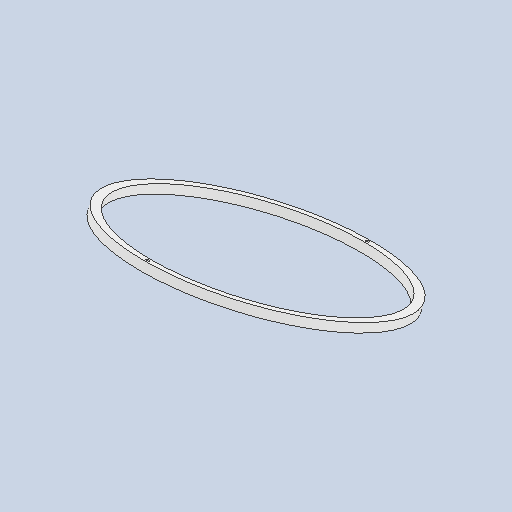
# Autodesk Inventor part: belt_liner_v2_Pom_r
Saved by Autodesk Inventor 2025.2 (Build 292293000, 293)
## iProperties
Created: 2025-01-06
Part Number: belt_liner_v2_Pom_r
Material: ABS プラスチック
Document SubType Name: Modeling
Designer: haruy
Density: 1.06 g/cm^3
Appearance: 白
Author: haruy
Autodesk Inventor part; units mm, degrees
ref_plane "YZ Plane" through (0, 0, 0) normal (1, 0, 0) x (0, 1, 0)
ref_plane "XZ Plane" through (0, 0, 0) normal (0, 1, 0) x (-1, 0, 0)
ref_plane "XY Plane" through (0, 0, 0) normal (0, 0, 1) x (1, 0, 0)
derived "belt_liner_v2_Sketch_Base.ipt"
sketch "スケッチ1" plane through (300, 0, 0) normal (1, 0, 0) x (0, 1, 0)
  circle A0 centre (0, 0) radius 23.875
  circle A1 centre (981.994578, -416.831968) radius 23.875 construction
  line L0 (0, 0) -> (0, -985.832038)
  line L1 (0.888552, 67.547515) -> (6.749519, 81.355087)
  line L2 (6.749519, 81.355087) -> (503.82214, -129.639722)
  line L3 (503.82214, -129.639722) -> (497.961173, -143.447295)
  line L4 (497.961173, -143.447295) -> (0.888552, 67.547515)
  line L5 (0, 0) -> (981.994578, -416.831968)
  line L6 (-41.329946, -31.913035) -> (-47.190913, -45.720608)
  line L7 (-47.190913, -45.720608) -> (953.397863, -470.445344)
  line L8 (953.397863, -470.445344) -> (959.258829, -456.637772)
  line L9 (959.258829, -456.637772) -> (-41.329946, -31.913035)
  line L10 (11.023029, 79.54109) -> (11.023029, 79.54109)
  line L11 (0.888552, 67.547515) -> (82.443045, 32.929686)
  line L12 (82.443045, 32.929686) -> (80.489389, 28.327162)
  line L13 (80.489389, 28.327162) -> (-1.065103, 62.94499)
  line L14 (-1.065103, 62.94499) -> (0.888552, 67.547515)
  line L15 (497.961173, -143.447295) -> (479.780011, -135.729849)
  line L16 (0, -985.832038) -> (0, 0)
  circle A2 centre (0, 0) radius 12.5
  circle A3 centre (0, 0) radius 15
  line L17 (0, 0) -> (0, 0)
  circle A4 centre (0, 0) radius 25.575 construction
  line L18 (0, 0) -> (0, 0)
  line L19 (0, 0) -> (0, 0)
  line L20 (-41.329946, -31.913035) -> (-39.376291, -27.310511)
  line L21 (-39.376291, -27.310511) -> (35.045481, -58.900678)
  line L22 (39.535359, -66.23832) -> (-41.329946, -31.913035)
  line L23 (84.992432, 48.142941) -> (503.82214, -129.639722)
  line L24 (503.82214, -129.639722) -> (505.971161, -124.576945)
  circle A5 centre (981.994578, -416.831968) radius 5
  line L25 (959.258829, -456.637772) -> (931.643684, -444.915838)
  line L26 (931.643684, -444.915838) -> (933.597339, -440.313313)
  line L27 (933.597339, -440.313313) -> (961.212485, -452.035247)
  line L28 (961.212485, -452.035247) -> (959.258829, -456.637772)
  circle A6 centre (977.392053, -414.878312) radius 5.1
  line L29 (981.994578, -416.831968) -> (543.18707, -230.569232)
  circle A7 centre (1000.404675, -424.64659) radius 5.1
  line L30 (979.384782, -410.183737) -> (1002.397403, -419.952016)
  line L31 (975.399325, -419.572887) -> (998.411946, -429.341165)
  circle A8 centre (981.994578, -416.831968) radius 22.175 construction
  line L32 (1033.115714, -370.60692) -> (1016.705007, -409.268124)
  line L33 (1016.705007, -409.268124) -> (1025.910055, -413.175435)
  line L34 (1025.910055, -413.175435) -> (1042.320763, -374.514232)
  line L35 (1042.320763, -374.514232) -> (1033.115714, -370.60692)
  circle A9 centre (977.392053, -414.878312) radius 10.1 construction
  circle A10 centre (1000.404675, -424.64659) radius 10.1 construction
  line L36 (981.338438, -405.581213) -> (1004.351059, -415.349491) construction
  line L37 (973.445669, -424.175411) -> (996.45829, -433.943689) construction
  line L38 (981.338438, -405.581213) -> (970.226961, -400.864671) construction
  line L39 (968.094954, -410.931928) -> (972.041339, -401.634829) construction
  line L40 (1004.351059, -415.349491) -> (1013.197672, -419.104656) construction
  line L41 (1013.197672, -419.104656) -> (1013.556108, -419.256803)
  line L42 (82.443045, 32.929686) -> (80.489389, 28.327162)
  line L43 (80.489389, 28.327162) -> (103.412197, 18.597007)
  line L44 (103.412197, 18.597007) -> (105.365853, 23.199531)
  line L45 (105.365853, 23.199531) -> (82.443045, 32.929686)
  line L46 (-47.190913, -45.720608) -> (-47.190913, -625.255323)
  line L47 (996.45829, -433.943689) -> (1004.351059, -415.349491)
  line L48 (1004.351059, -415.349491) -> (1013.556108, -419.256803)
  line L49 (1013.556108, -419.256803) -> (1005.663339, -437.851001)
  line L50 (1005.663339, -437.851001) -> (996.45829, -433.943689) construction
  line L51 (503.82214, -129.639722) -> (497.961173, -143.447295)
  line L52 (497.961173, -143.447295) -> (1139.553056, -415.786891)
  line L53 (1139.553056, -415.786891) -> (1145.414023, -401.979319)
  line L54 (1145.414023, -401.979319) -> (503.82214, -129.639722)
  line L55 (-12.338478, -2.002986) -> (-33.38334, -51.581575)
  line L56 (-12.338478, -2.002986) -> (20.557092, 75.49412)
  circle A11 centre (36.731918, 49.617007) radius 1.5
  circle A12 centre (59.74454, 39.848729) radius 1.5
  circle A13 centre (951.030609, -450.429198) radius 1.5
  circle A14 centre (0, 0) radius 45
  circle A15 centre (59.875702, 3.860095) radius 22 construction
  circle A16 centre (59.875702, 3.860095) radius 15
  circle A17 centre (92.92231, 14.358817) radius 3
  circle A18 centre (50.87986, -21.597219) radius 3
  circle A19 centre (50.87986, -21.597219) radius 4 construction
  circle A20 centre (38.816438, -45.752422) radius 22 construction
  circle A21 centre (38.816438, -45.752422) radius 15
  circle A22 centre (50.87986, -21.597219) radius 3
  line L57 (63.127818, -76.307043) -> (65.081474, -71.704519)
  line L58 (103.412197, 18.597007) -> (65.081474, -71.704519)
  circle A23 centre (82.757161, 30.080451) radius 1.5
  circle A24 centre (981.994578, -416.831968) radius 6 construction
  circle A25 centre (0, 0) radius 25.575 construction
  circle A26 centre (0, 0) radius 25.525
  circle A27 centre (981.994578, -416.831968) radius 25.525
  line L59 (991.96799, -393.336081) -> (9.973412, 23.495886)
  circle A28 centre (964.412935, -409.369003) radius 4
  circle A29 centre (964.412935, -409.369003) radius 1.5
  circle A30 centre (981.994578, -416.831968) radius 18.525 construction
  circle A31 centre (987.166133, -404.904478) radius 4
  line L60 (978.140244, -426.16814) -> (982.086628, -416.871041)
  circle A32 centre (987.166133, -404.904478) radius 1.5
  line L61 (972.041339, -401.634829) -> (974.737384, -395.283345) construction
  line L62 (974.737384, -395.283345) -> (1016.252152, -412.905319)
  line L63 (1013.556108, -419.256803) -> (1016.252152, -412.905319)
  line L64 (974.737384, -395.283345) -> (961.814136, -406.328239)
  line L65 (961.452525, -426.58051) -> (1002.967294, -444.202484)
  line L66 (961.452525, -426.58051) -> (960.420315, -409.611876)
  line L67 (1005.663339, -437.851001) -> (1002.967294, -444.202484)
  circle A33 centre (977.007123, -428.837604) radius 4
  circle A34 centre (977.007123, -428.837604) radius 1.5
  circle A35 centre (294.226959, 105.986805) radius 120
  line L68 (111.935344, -6.748062) -> (102.730296, -2.84075) construction
  line L69 (1139.553056, -415.786891) -> (1111.93791, -404.064958)
  line L70 (1111.93791, -404.064958) -> (1109.984255, -408.667482)
  line L71 (1109.984255, -408.667482) -> (1137.5994, -420.389416)
  line L72 (1137.5994, -420.389416) -> (1139.553056, -415.786891)
  circle A36 centre (1129.37118, -414.180842) radius 1.5
  line L73 (103.412197, 18.597007) -> (105.365853, 23.199531)
  line L74 (105.365853, 23.199531) -> (115.951659, 18.706124)
  line L75 (115.951659, 18.706124) -> (113.998003, 14.103599)
  line L76 (113.998003, 14.103599) -> (103.412197, 18.597007)
  circle A37 centre (1120.166131, -410.273531) radius 1.5
  circle A38 centre (941.82556, -446.521887) radius 1.5
  line L77 (35.045481, -58.900678) -> (65.10101, -71.658494)
  line L78 (503.82214, -129.639722) -> (505.971161, -124.576945)
  line L79 (122.594088, 34.354706) -> (184.728166, 7.980355)
  line L80 (184.728166, 7.980355) -> (186.681821, 12.582879)
  line L81 (186.681821, 12.582879) -> (124.547744, 38.95723)
  line L82 (124.547744, 38.95723) -> (122.594088, 34.354706)
  circle A39 centre (136.696474, 38.145842) radius 4
  circle A40 centre (136.696474, 38.145842) radius 11
  circle A41 centre (164.31162, 26.423908) radius 4
  circle A42 centre (164.31162, 26.423908) radius 11
  line L83 (134.517527, 22.775344) -> (131.782409, 16.33181)
  line L84 (131.782409, 16.33181) -> (152.033515, 7.735726)
  line L85 (152.033515, 7.735726) -> (154.768633, 14.17926)
  line L86 (154.768633, 14.17926) -> (134.517527, 22.775344)
  line L87 (144.64308, 18.477302) -> (141.907962, 12.033768)
  line L88 (162.132672, 11.053411) -> (159.397554, 4.609877)
  line L89 (159.397554, 4.609877) -> (179.648661, -3.986208)
  line L90 (179.648661, -3.986208) -> (182.383779, 2.457326)
  line L91 (182.383779, 2.457326) -> (162.132672, 11.053411)
  line L92 (172.258225, 6.755368) -> (169.523108, 0.311834)
  line L93 (3.819036, 74.451301) -> (1142.483539, -408.883105)
  line L94 (177.304274, -9.509237) -> (175.350619, -14.111762)
  line L95 (115.170197, 16.865114) -> (177.304274, -9.509237)
  line L96 (175.350619, -14.111762) -> (113.216541, 12.26259)
  line L97 (113.216541, 12.26259) -> (115.170197, 16.865114)
  circle A43 centre (122.239422, 4.087162) radius 11
  circle A44 centre (122.239422, 4.087162) radius 4
  circle A45 centre (149.854568, -7.634772) radius 11
  circle A46 centre (149.854568, -7.634772) radius 4
  line L98 (143.305447, 25.563256) -> (150.669486, 22.437407)
  line L99 (150.669486, 22.437407) -> (143.245595, 4.947814)
  line L100 (143.245595, 4.947814) -> (135.881556, 8.073663)
  line L101 (135.881556, 8.073663) -> (143.305447, 25.563256)
  line L102 (170.920593, 13.841322) -> (178.284632, 10.715473)
  line L103 (178.284632, 10.715473) -> (170.86074, -6.774119)
  line L104 (170.86074, -6.774119) -> (163.496701, -3.64827)
  line L105 (163.496701, -3.64827) -> (170.920593, 13.841322)
  line L106 (113.216541, 12.26259) -> (99.540951, -19.95508)
  line L107 (99.540951, -19.95508) -> (108.746, -23.862392)
  line L108 (108.746, -23.862392) -> (122.421589, 8.355278)
  line L109 (122.421589, 8.355278) -> (113.216541, 12.26259)
  line L110 (113.216541, 12.26259) -> (150.95724, -3.757387)
  line L111 (150.95724, -3.757387) -> (147.831391, -11.121426)
  line L112 (147.831391, -11.121426) -> (110.090692, 4.898551)
  line L113 (110.090692, 4.898551) -> (113.216541, 12.26259)
  line L114 (133.9279, 3.471139) -> (141.291939, 0.34529)
  line L115 (141.291939, 0.34529) -> (140.119746, -2.416224)
  line L116 (140.119746, -2.416224) -> (132.755707, 0.709625)
  line L117 (132.755707, 0.709625) -> (133.9279, 3.471139)
  circle A47 centre (60.86282, -61.168606) radius 3
  circle A48 centre (-3.532924, -45.241018) radius 1.25
  circle A49 centre (19.479697, -55.009296) radius 1.25
  circle A50 centre (42.492318, -64.777574) radius 1.25
  circle A51 centre (294.226959, 105.986805) radius 130
  line L118 (294.226959, 105.986805) -> (183.766377, 152.87454)
  line L119 (294.226959, 105.986805) -> (182.964897, 61.034014)
  line L120 (294.226959, 105.986805) -> (249.274168, 217.248867)
  line L121 (251.618555, 222.771896) -> (180.62051, 55.510984)
  line L122 (180.62051, 55.510984) -> (175.097481, 57.855371)
  line L123 (175.097481, 57.855371) -> (246.095526, 225.116283)
  line L124 (246.095526, 225.116283) -> (251.618555, 222.771896)
  line L125 (294.226959, 105.986805) -> (243.431912, -13.678826)
  line L126 (1032.334252, -372.44793) -> (1030.380596, -377.050454)
  line L127 (1030.380596, -377.050454) -> (1092.514674, -403.424805)
  line L128 (1092.514674, -403.424805) -> (1094.46833, -398.822281)
  line L129 (1094.46833, -398.822281) -> (1032.334252, -372.44793)
  line L130 (1094.46833, -398.822281) -> (1092.514674, -403.424805)
  line L131 (1092.514674, -403.424805) -> (1109.202792, -410.508491)
  line L132 (1109.202792, -410.508491) -> (1111.156448, -405.905967)
  line L133 (1111.156448, -405.905967) -> (1094.46833, -398.822281)
  line L134 (974.737384, -395.283345) -> (1109.984255, -408.667482)
  circle A52 centre (981.994578, -416.831968) radius 35.525
  line L135 (1103.309517, -408.006945) -> (1106.044635, -401.563411)
  circle A53 centre (982.086628, -416.871041) radius 8.5
  line L136 (221.076402, 266.364498) -> (113.216541, 12.26259)
  line L137 (256.70736, -7.996877) -> (252.787465, -17.231572)
  line L138 (252.787465, -17.231572) -> (175.350619, -14.111762)
  line L139 (180.62051, 55.510984) -> (201.09616, 30.312145)
  line L140 (246.095526, 225.116283) -> (246.927704, 227.076773)
  circle A54 centre (128.17344, 34.702313) radius 1.5
  circle A55 centre (181.102469, 12.235273) radius 1.5
  circle A56 centre (118.795893, 12.610196) radius 1.5
  circle A57 centre (171.724922, -9.856844) radius 1.5
  line L141 (175.097481, 57.855371) -> (177.441867, 63.3784)
  line L142 (177.441867, 63.3784) -> (172.839343, 65.332056)
  line L143 (172.839343, 65.332056) -> (170.494956, 59.809027)
  line L144 (170.494956, 59.809027) -> (175.097481, 57.855371)
  line L145 (246.095526, 225.116283) -> (243.751139, 219.593254)
  line L146 (243.751139, 219.593254) -> (239.148614, 221.54691)
  line L147 (239.148614, 221.54691) -> (241.493001, 227.069939)
  line L148 (241.493001, 227.069939) -> (246.095526, 225.116283)
  circle A58 centre (242.62207, 223.331597) radius 1.5
  line L149 (246.927704, 227.076773) -> (241.493001, 227.069939)
  line L150 (241.493001, 227.069939) -> (222.121536, 214.157078)
  circle A59 centre (173.968412, 61.593714) radius 1.5
  line L151 (249.274168, 217.248867) -> (243.751139, 219.593254)
  line L152 (182.964897, 61.034014) -> (177.441867, 63.3784)
  line L153 (1137.5994, -420.389416) -> (959.258829, -456.637772)
  line L154 (933.597339, -440.313313) -> (961.332007, -406.817948)
  line L155 (1111.93791, -404.064958) -> (1109.984255, -408.667482)
  line L156 (1109.984255, -408.667482) -> (1102.620216, -405.541633)
  line L157 (1102.620216, -405.541633) -> (1104.573871, -400.939108)
  line L158 (1104.573871, -400.939108) -> (1111.93791, -404.064958)
  line L159 (-29.856643, -31.747305) -> (-44.856643, -31.747305)
  line L160 (-44.856643, -31.747305) -> (-44.856643, -284.247305)
  line L161 (-44.856643, -284.247305) -> (-29.856643, -284.247305)
  line L162 (-29.856643, -284.247305) -> (-29.856643, -31.747305)
  line L163 (471.143357, -269.247305) -> (-44.856643, -269.247305)
  line L164 (-44.856643, -269.247305) -> (-44.856643, -284.247305)
  line L165 (-44.856643, -284.247305) -> (471.143357, -284.247305)
  line L166 (471.143357, -284.247305) -> (471.143357, -269.247305)
  line L167 (-14.973243, -59.396197) -> (-9.112276, -45.588624)
  line L168 (12.641902, -71.118131) -> (18.502869, -57.310558)
  line L169 (-44.856643, -78.747305) -> (-67.856643, -78.747305)
  line L170 (-67.856643, -78.747305) -> (-67.856643, -138.747305)
  line L171 (-67.856643, -138.747305) -> (-44.856643, -138.747305)
  line L172 (-44.856643, -138.747305) -> (-44.856643, -78.747305)
  line L173 (-44.856643, -98.747305) -> (-89.856643, -98.747305)
  line L174 (-89.856643, -98.747305) -> (-89.856643, -118.747305)
  line L175 (-89.856643, -118.747305) -> (-44.856643, -118.747305)
  line L176 (-44.856643, -118.747305) -> (-44.856643, -98.747305)
  line L177 (-29.856643, -78.747305) -> (-44.856643, -78.747305)
  line L178 (-89.856643, -108.747305) -> (-44.856643, -108.747305)
  line L179 (-53.856643, -248.747305) -> (-58.856643, -248.747305)
  line L180 (-58.856643, -248.747305) -> (-58.856643, -258.747305)
  line L181 (-58.856643, -258.747305) -> (-53.856643, -258.747305)
  line L182 (-53.856643, -258.747305) -> (-53.856643, -248.747305)
  line L183 (-44.856643, -240.248994) -> (-49.856643, -240.248994)
  line L184 (-49.856643, -240.248994) -> (-49.856643, -266.157001)
  line L185 (-49.856643, -266.157001) -> (-44.856643, -266.157001)
  line L186 (-44.856643, -266.157001) -> (-44.856643, -240.248994)
  line L187 (-47.356643, -240.248994) -> (-47.356643, -266.157001)
  line L188 (441.143357, -269.247305) -> (441.143357, -284.247305)
  line L189 (471.143357, -284.247305) -> (514.74277, -284.247305)
  line L190 (514.74277, -284.247305) -> (520.603737, -270.439732)
  line L191 (471.143357, -269.247305) -> (479.404985, -269.247305)
  line L192 (479.404985, -269.247305) -> (485.265952, -255.439732)
  line L193 (-58.856643, -253.747305) -> (-53.856643, -253.747305)
  line L194 (-85.856643, 246.112358) -> (-105.856643, 246.112358)
  line L195 (-105.856643, 246.112358) -> (-105.856643, -703.706588)
  line L196 (-105.856643, -703.706588) -> (-85.856643, -703.706588)
  line L197 (-85.856643, -703.706588) -> (-85.856643, 246.112358)
  line L198 (242.62207, 223.331597) -> (-85.856643, 223.331597)
  line L199 (-23.79201, -270.027244) -> (-25.593912, -279.863562)
  line L200 (-25.593912, -279.863562) -> (928.443519, -454.632373)
  line L201 (928.443519, -454.632373) -> (930.245421, -444.796055)
  line L202 (930.245421, -444.796055) -> (-23.79201, -270.027244)
  point P0 (50.87986, -21.597219)
  point P1 (81.466217, 30.628424)
  point P2 (249.274168, 217.248867)
  point P3 (-27.522373, -37.774002)
  point P4 (-37.356643, -41.747305)
  point P5 (-37.356643, -276.747305)
  point P6 (461.143357, -276.747305)
  point P7 (451.143357, -276.747305)
  point P8 (491.933647, -266.417704)
  point P9 (501.138696, -270.325015)
  point P10 (-14.856643, -276.747305)
  point P11 (919.508152, -447.912313)
revolve "回転1" add sketch "スケッチ1" angle 360 about axis through (300, 294.226959, 105.986805) along (0, -0.9205049, 0.3907311) contours L124 L121 L151 L123
sketch "スケッチ2" plane through (300, 216.119532, 139.14144) normal (0, 0.9205049, -0.3907311) x (1, 0, 0)
  circle A0 centre (0, 0) radius 84.852814
  circle A1 centre (0, 0) radius 84.852814
  circle A2 centre (0, 0) radius 87.852814
  point P0 (-300, 212.525)
  point P1 (0, -87.852814)
  point P2 (0, 87.852814)
  dimension "d2" = 3
  dimension "d4" = 0
  dimension "d5" = 0
  constraints: 2 centre point, 2 point on circle, 1 coincident
  measures "d2" radial gap between concentric circles of A0 A2
  measures "d4" horizontal distance of A1.centre A2.start
  measures "d5" horizontal distance of A1.centre A2.end
hole "穴1" at (300, 250.446361, 220.010382) at (300, 181.792703, 58.272499) direction (0, -0.9205049, 0.3907311) diameter 2.5 end through all
